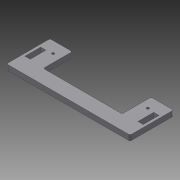
# Autodesk Inventor part: Mount_LCD_Back
Saved by Autodesk Inventor 2014 (Build 180170000, 170)
## iProperties
Created: 2014-10-26
Part Number: Mount_LCD_Back
Material: Generic
Document SubType Name: Modeling
Designer: ThatOtherGuy
Density: 1 g/cm^3
Appearance: Default
Author: ThatOtherGuy
Autodesk Inventor part; units mm, degrees
ref_plane "YZ Plane" through (0, 0, 0) normal (1, 0, 0) x (0, 1, 0)
ref_plane "XZ Plane" through (0, 0, 0) normal (0, 1, 0) x (-1, 0, 0)
ref_plane "XY Plane" through (0, 0, 0) normal (0, 0, 1) x (1, 0, 0)
sketch "Sketch1" plane through (0, 0, 0) normal (0, 0, 1) x (1, 0, 0)
  line L0 (0, 0) -> (156.5, 0)
  line L1 (156.5, 0) -> (156.5, 55)
  line L2 (156.5, 55) -> (0, 55)
  line L3 (0, 55) -> (0, 0)
  line L4 (3.269, 40) -> (10, 40)
  line L5 (10, 40) -> (10, 20)
  line L6 (10, 20) -> (3.269, 20)
  line L7 (3.269, 20) -> (3.269, 40)
  line L8 (146.5, 40) -> (153.231, 40)
  line L9 (153.231, 40) -> (153.231, 20)
  line L10 (153.231, 20) -> (146.5, 20)
  line L11 (146.5, 20) -> (146.5, 40)
  line L12 (68.25, 10) -> (88.25, 10)
  line L13 (88.25, 10) -> (88.25, 3.269)
  line L14 (88.25, 3.269) -> (68.25, 3.269)
  line L15 (68.25, 3.269) -> (68.25, 10)
  line L16 (28.25, 55) -> (128.25, 55)
  line L17 (128.25, 55) -> (128.25, 18.269)
  line L18 (128.25, 18.269) -> (28.25, 18.269)
  line L19 (28.25, 18.269) -> (28.25, 55)
  point P0 (3.269, 30)
  point P1 (153.231, 30)
  point P2 (78.25, 18.269)
  point P3 (78.25, 55)
  dimension "d0" = 55
  dimension "d1" = 156.5
  dimension "d2" = 136.5
  dimension "d3" = 6.731
  dimension "d4" = 58.25
  dimension "d5" = 58.25
  dimension "d6" = 20
  dimension "d7" = 3.269
  dimension "d8" = 3.269
  dimension "d25" = 10
  dimension "d26" = 10
  dimension "d28" = 36.731
  dimension "d29" = 100
  constraints: 40 end point, 10 parallel, 5 horizontal, 5 perpendicular, 4 equal length, 4 midpoint, 1 horizontal alignment, 1 point on line, 1 vertical alignment
  measures "d0" distance of L2.end L0.start
  measures "d1" distance of L1.end L2.end
  measures "d2" distance between parallel lines of L11 L5
  measures "d3" distance of L4.start L4.end
  measures "d4" distance between parallel lines of L15 L5
  measures "d5" distance between parallel lines of L11 L13
  measures "d6" distance of L12.start L12.end
  measures "d7" distance between parallel lines of L3 L7
  measures "d8" distance between parallel lines of L1 L9
  measures "d25" distance between parallel lines of L0 L12
  measures "d26" distance between parallel lines of L12 L6
  measures "d28" distance of L18.end L16.start
  measures "d29" distance of L17.end L18.end
extrude "Extrusion1" add sketch "Sketch1" along normal blind 6.731 contours L3 L2 L19 L18 L17 L1 L0 | L12 L13 L14 L15
sketch "Sketch2" plane through (0, 0, 6.731) normal (0, 0, 1) x (1, 0, 0)
  line L0 (10, 40) -> (10, 20) projected
  line L1 (156.5, 55) -> (0, 55) projected
  line L2 (146.5, 20) -> (146.5, 40) projected
  point P0 (18.25, 40.769)
  point P1 (138.25, 40.769)
  dimension "d14" = 120
  dimension "d15" = 14.231
  dimension "d16" = -8.25
  dimension "d30" = -8.25
  constraints: 1 horizontal alignment
  measures "d14" distance of point (138.25, 40.769) point (18.25, 40.769)
  measures "d15" distance from line of L1 point (18.25, 40.769)
  measures "d16" distance from line of L0 point (18.25, 40.769)
  measures "d30" distance from line of L2 point (138.25, 40.769)
hole "Hole1" at (18.25, 40.769, 6.731) at (138.25, 40.769, 6.731) direction (0, 0, -1) diameter 3.176 end through all
fillet "Fillet1" radius 2 8 edges at (156.5, 55, 3.3655) (0, 55, 3.3655) (0, 0, 3.3655) (156.5, 0, 3.3655) (28.25, 18.269, 3.3655) (28.25, 55, 3.3655) (128.25, 55, 3.3655) (128.25, 18.269, 3.3655)
equation "\"d3\" = THICKB"
equation "\"d4\" = d5"
equation "\"d7\" = d8"
equation "\"d12\" = THICKB"
equation "\"d16\" = d30"
equation "\"THICKA\" = 3.175"
equation "\"THICKB\" = 6.731"
equation "\"THICKC\" = 12.7"
equation "\"THICKPLY\" = 5"
equation "\"MAGDIA\" = 9.5"
equation "\"BALLDIA\" = 12"
body "Solid1"
